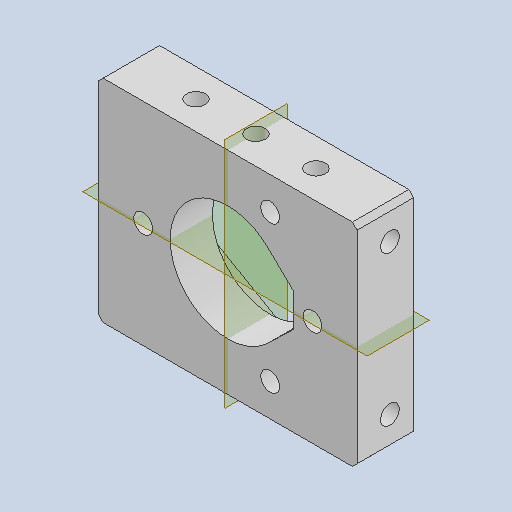
# Autodesk Inventor part: Mount Side
Saved by Autodesk Inventor 2022 (Build 260153000, 153)
## iProperties
Created: 2022-08-19
Part Number: Mount Side
Material: Generic
Document SubType Name: Modeling
Designer: Nick
Density: 1 g/cm^3
Appearance: Default
Mass: 21.3325 g
Surface Area: 83.7713 cm^2
Volume: 21.3325 cm^3
Author: Nick
Autodesk Inventor part; units mm, degrees
ref_plane "YZ Plane" through (0, 0, 0) normal (1, 0, 0) x (0, 1, 0)
ref_plane "XZ Plane" through (0, 0, 0) normal (0, 1, 0) x (-1, 0, 0)
ref_plane "XY Plane" through (0, 0, 0) normal (0, 0, 1) x (1, 0, 0)
sketch "Sketch1" plane through (0, 0, 0) normal (0, 0, 1) x (1, 0, 0)
  line L0 (0, 0) -> (55, 0)
  line L1 (55, 0) -> (55, 45)
  line L2 (55, 45) -> (0, 45)
  line L3 (0, 45) -> (0, 0)
  circle A0 centre (27.5, 22.5) radius 12.25
  line L4 (36.0177, 31.304) -> (41.5, 26)
  line L5 (41.5, 26) -> (41.5, 19)
  line L6 (41.5, 19) -> (36.0177, 13.696)
  circle A1 centre (27.5, 22.5) radius 8 construction
  line L7 (8.5, 27.6962) -> (32.5, 41.5526)
  line L8 (41.5, 36.3564) -> (41.5, 8.6436)
  line L9 (32.5, 3.4474) -> (8.5, 17.3038)
  arc A2 (41.5, 36.3564) -> (32.5, 41.5526) centre (35.5, 36.3564) ccw
  arc A3 (8.5, 27.6962) -> (8.5, 17.3038) centre (11.5, 22.5) ccw
  arc A4 (32.5, 3.4474) -> (41.5, 8.6436) centre (35.5, 8.6436) ccw
  line L10 (27.5, 22.5) -> (36.5, 6.9115) construction
  line L11 (27.5, 22.5) -> (9.5, 22.5) construction
  line L12 (27.5, 22.5) -> (36.5, 38.0885) construction
  point P0 (55, 22.5)
  point P1 (27.5, 45)
  point P2 (41.5, 22.5)
  point P3 (-0.5, 22.5)
  point P4 (41.5, 46.7487)
  point P5 (41.5, -1.7487)
  dimension "d0" = 24.5
  dimension "d1" = 45
  dimension "d2" = 55
  dimension "d3" = 14
  dimension "d6" = 7
  dimension "d7" = 16
  dimension "d9" = 6
  dimension "d31" = 2
  dimension "d32" = 2
  dimension "d33" = 2
  constraints: 26 end point, 8 point on circle, 8 point on line, 8 tangent, 5 centre point, 3 midpoint, 2 coincident, 2 equal radius, 2 horizontal, 2 horizontal alignment, 2 parallel, 2 vertical, 1 collinear, 1 perpendicular, 1 vertical alignment, 7 other
  measures "d0" diameter of A0
  measures "d1" distance of L0.end L1.end
  measures "d2" distance of L1.end L2.end
  measures "d3" distance from line of L5 A0.centre
  measures "d6" distance of L4.end L5.end
  measures "d7" diameter of A1
  measures "d9" radius of A2
  measures "d31" distance of A4.centre L10.end
  measures "d32" distance of A3.centre L11.end
  measures "d33" distance of A2.centre L12.end
extrude "Extrusion1" add sketch "Sketch1" along normal blind 12 contours L3 L2 L1 L0 | A0 L6 L8 A4 L9 A3 L7 A2 L4
extrude "Extrusion2" cut sketch "Sketch1" along normal blind 3 contours A0 L6 L8 A4 L9 A3 L7 A2 L4
hole "Hole1" at (36.5, 38.0885, 0) at (9.5, 22.5, 0) at (36.5, 6.9115, 0) direction (0, 0, 1) diameter 4 end through all
ref_plane "Work Plane1" through (27.5, 0, 0) normal (-1, 0, 0) x (0, 0, 1)
sketch "Sketch3" plane through (0, 0, 12) normal (0, 0, 1) x (1, 0, 0)
  circle A0 centre (45.5, 22.5) radius 1.8 projected
  point P0 (0, 0)
hole "Hole2" at (45.5, 22.5, 12) direction (0, 0, -1) diameter 4 end through all
sketch "Sketch4" plane through (2, 0, 0) normal (0, -1, 0) x (1, 0, 0)
  line L0 (-2, 12) -> (53, 12) projected
  line L1 (-2, 0) -> (53, 0) projected
  line L2 (53, 0) -> (53, 12) projected
  line L3 (-2, 0) -> (-2, 12) projected
  point P0 (38.25, 6)
  point P1 (25.5, 6)
  point P2 (12.75, 6)
  point P3 (0, 6)
  point P4 (25.5, 0)
  dimension "d35" = 12.75
  dimension "d36" = 12.75
  constraints: 3 horizontal alignment, 1 midpoint, 1 vertical alignment
  measures "d35" distance of point (25.5, 6) point (38.25, 6)
  measures "d36" distance of point (12.75, 6) point (25.5, 6)
hole "Hole3" at (40.25, 0, 6) at (27.5, 0, 6) at (14.75, 0, 6) direction (0, 1, 0) diameter 4 depth 5
ref_plane "Work Plane2" through (2, 22.5, 0) normal (0, -1, 0) x (1, 0, 0)
mirror "Mirror2" about plane through (2, 22.5, 0) normal (0, -1, 0) of "Hole3"
chamfer "Chamfer1" distance 1 angle 45 4 edges at (0, 45, 6) (0, 0, 6) (55, 0, 6) (55, 45, 6)
sketch "Sketch5" plane through (55, 1, 0) normal (1, 0, 0) x (0, 0, -1)
  circle A0 centre (-5.03, 5.5969) radius 1.7018
  circle A1 centre (-5, 37.4031) radius 1.7018
  point P0 (0, -1)
  constraints: 2 centre point, 4 other
hole "Hole4" at (55, 6.5969, 5.03) at (55, 38.4031, 5) direction (-1, 0, 0) diameter 4 depth 8
equation "\"d31\" = d32"
equation "\"d32\" = d33"
equation "\"d35\" = d37"
equation "\"d36\" = d37"
equation "\"d37\" = 12.75"
body "Solid1"
